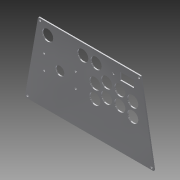
# Autodesk Inventor part: Panel_top
Saved by Autodesk Inventor 2013 (Build 170138000, 138)
## iProperties
Created: 2012-07-09
Part Number: Panel_top
Material: Aluminum 1100-H18
Document SubType Name: Modeling
Designer: mstine
Density: 1 g/cm^3
Author: mstine
Autodesk Inventor part; units mm, degrees
ref_plane "YZ Plane" through (0, 0, 0) normal (1, 0, 0) x (0, 1, 0)
ref_plane "XZ Plane" through (0, 0, 0) normal (0, 1, 0) x (-1, 0, 0)
ref_plane "XY Plane" through (0, 0, 0) normal (0, 0, 1) x (1, 0, 0)
sketch "Sketch1" plane through (0, 0, 0) normal (0, 0, 1) x (1, 0, 0)
  circle A0 centre (-80, 0) radius 12
  circle A1 centre (15, -18) radius 15
  circle A2 centre (15, 18) radius 15
  circle A3 centre (46.25, 0) radius 15
  circle A4 centre (46.25, 36) radius 15
  circle A5 centre (82.25, 0) radius 15
  circle A6 centre (82.25, 36) radius 15
  circle A7 centre (117.25, -9) radius 15
  circle A8 centre (117.25, 27) radius 15
  line L0 (-175, -108) -> (175, -108)
  line L1 (-175, -108) -> (-138.853, 97)
  line L2 (175, -108) -> (138.853, 97)
  line L3 (-138.853, 97) -> (138.853, 97)
  line L4 (46.25, 36) -> (82.25, 36) construction
  line L5 (82.25, 36) -> (82.25, 0) construction
  line L6 (46.25, 36) -> (46.25, 0) construction
  line L7 (46.25, 0) -> (82.25, 0) construction
  line L8 (117.25, 27) -> (117.25, -9) construction
  line L9 (15, 18) -> (15, -18) construction
  circle A9 centre (18, 67) radius 15
  circle A10 centre (-18, 67) radius 15
  circle A11 centre (-113, 67) radius 15
  line L10 (83, 79) -> (121, 79)
  line L11 (121, 79) -> (121, 59.7)
  line L12 (121, 59.7) -> (83, 59.7)
  line L13 (83, 59.7) -> (83, 79)
  line L14 (0, 97) -> (0, -108) construction
  point P0 (0, 0)
  point P1 (-167.8495, -102)
  point P2 (-133.8184, 91)
  point P3 (167.8495, -102)
  point P4 (133.8184, 91)
  point P5 (-122.5, -20.25)
  point P6 (-37.5, -20.25)
  point P7 (-122.5, 20.25)
  point P8 (-37.5, 20.25)
  dimension "d3" = 24
  dimension "d18" = 30
  dimension "d37" = 90
  dimension "d38" = 80
  dimension "d40" = 80
  dimension "d42" = 350
  dimension "d45" = 31.25
  dimension "d46" = 36
  dimension "d47" = 35
  dimension "d48" = 18
  dimension "d49" = 18
  dimension "d50" = 18
  dimension "d51" = 9
  dimension "d52" = 27
  dimension "d53" = 95
  dimension "d57" = 205
  dimension "d58" = 160
  dimension "d65" = 19.3
  dimension "d66" = 38
  dimension "d67" = 30
  dimension "d73" = 30
  dimension "d74" = 36
  dimension "d76" = 18
  dimension "d77" = 95
  dimension "d78" = 18
  dimension "d79" = 65
  dimension "d92" = 6
  dimension "d93" = 6
  dimension "d94" = 6
  dimension "d95" = 6
  dimension "d96" = 20.25
  dimension "d102" = 42.5
  dimension "d103" = 85
  dimension "d104" = 40.5
  constraints: 30 end point, 12 centre point, 9 equal radius, 7 horizontal alignment, 7 vertical alignment, 6 parallel, 4 perpendicular, 2 coincident, 2 horizontal, 2 midpoint, 2 symmetric about line
  measures "d3" diameter of A0
  measures "d18" diameter of A8
  measures "d37" distance from line of L0 L9.end
  measures "d38" angle of L0 L1
  measures "d40" angle of L0 L2
  measures "d42" distance of L0.start L0.end
  measures "d45" horizontal distance of L6.end L9.end
  measures "d46" distance of L5.end L6.end
  measures "d47" horizontal distance of L8.end L5.end
  measures "d48" vertical distance of L6.end L9.end
  measures "d49" vertical distance of L9.start L4.start
  measures "d50" vertical distance of point (0, 0) L9.start
  measures "d51" vertical distance of L8.end L5.end
  measures "d52" vertical distance of point (0, 0) L8.start
  measures "d53" horizontal distance of A0.centre L9.start
  measures "d57" vertical distance of L0.start L1.end
  measures "d58" horizontal distance of L0.end L9.end
  measures "d65" distance between parallel lines of L12 L10
  measures "d66" distance between parallel lines of L11 L13
  measures "d67" diameter of A10
  measures "d73" distance from line of L3 A10.centre
  measures "d74" distance of A9.centre A10.centre
  measures "d76" horizontal distance of point (0, 97) A9.centre
  measures "d77" distance of A10.centre A11.centre
  measures "d78" distance between parallel lines of L3 L10
  measures "d79" distance from line of L13 A9.centre
  measures "d92" distance from line of L0 point (-167.849, -102)
  measures "d93" distance from line of L1 point (-167.849, -102)
  measures "d94" distance from line of L1 point (-133.818, 91)
  measures "d95" distance from line of point (-133.818, 91) L3
  measures "d96" vertical distance of A0.centre point (-122.5, -20.25)
  measures "d102" horizontal distance of A0.centre point (-122.5, -20.25)
  measures "d103" distance of point (-37.5, -20.25) point (-122.5, -20.25)
  measures "d104" distance of point (-122.5, -20.25) point (-122.5, 20.25)
extrude "Extrusion5" add sketch "Sketch1" against normal blind 3.175
hole "Hole1" at (-167.8495, -102, 0) at (-133.8184, 91, 0) at (133.8184, 91, 0) at (167.8495, -102, 0) at (-122.5, -20.25, 0) at (-37.5, -20.25, 0) at (-122.5, 20.25, 0) at (-37.5, 20.25, 0) direction (0, 0, -1) diameter 4 end through all countersink diameter 6 countersink angle 90
fillet "Fillet9" radius 2 1 edges at (-138.853, 97, -1.5875)
fillet "Fillet10" radius 2 1 edges at (-175, -108, -1.5875)
fillet "Fillet11" radius 2 1 edges at (175, -108, -1.5875)
fillet "Fillet12" radius 2 1 edges at (138.853, 97, -1.5875)
fillet "Fillet13" radius 0.5 1 edges at (83, 79, -1.5875)
fillet "Fillet14" radius 0.5 1 edges at (121, 79, -1.5875)
fillet "Fillet15" radius 0.5 1 edges at (121, 59.7, -1.5875)
fillet "Fillet16" radius 0.5 1 edges at (83, 59.7, -1.5875)
sketch "Sketch2" plane through (0, 0, -3.175) normal (0, 0, -1) x (-1, 0, 0)
  line L0 (-83, 78.5) -> (-83, 60.2) projected
  circle A0 centre (-18, 67) radius 15 projected
  point P0 (0, 0)
  point P1 (-65, 67)
  dimension "d130" = 18
  constraints: 1 horizontal alignment
  measures "d130" distance from line of L0 point (-65, 67)
hole "Hole3" at (65, 67, -3.175) direction (0, 0, 1) diameter 5.9 end through all counterbore diameter 9 counterbore depth 1.5875
body "Solid5"
